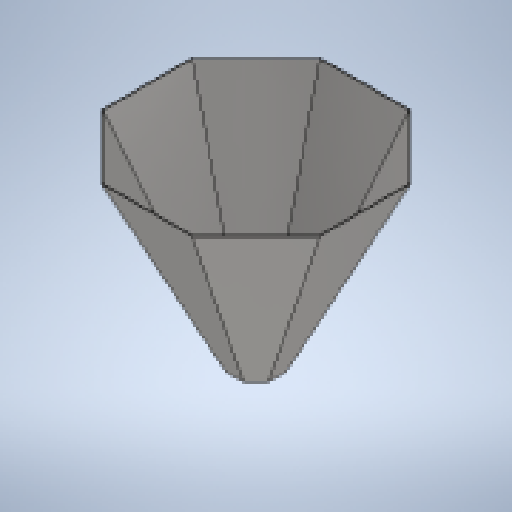
# Autodesk Inventor part: Funnel 1200x90 dummy
Saved by Autodesk Inventor 2025.1 (Build 291241020, 241B)
## iProperties
Created: 2025-07-11
Part Number: Funnel 1200x90 dummy
Material: Stainless Steel
Document SubType Name: Modeling
Designer: user
Density: 8 g/cm^3
Appearance: Semi-Polished
Author: user
Autodesk Inventor part; units mm, degrees
ref_plane "YZ Plane" through (0, 0, 0) normal (1, 0, 0) x (0, 1, 0)
ref_plane "XZ Plane" through (0, 0, 0) normal (0, 1, 0) x (-1, 0, 0)
ref_plane "XY Plane" through (0, 0, 0) normal (0, 0, 1) x (1, 0, 0)
sketch "Sketch1" plane through (0, 0, 0) normal (0, 0, 1) x (1, 0, 0)
  line L0 (18.6396, 45) -> (45, 18.6396)
  line L1 (45, 18.6396) -> (45, -18.6396)
  line L2 (45, -18.6396) -> (18.6396, -45)
  line L3 (18.6396, -45) -> (-18.6396, -45)
  line L4 (-18.6396, -45) -> (-45, -18.6396)
  line L5 (-45, -18.6396) -> (-45, 18.6396)
  line L6 (-45, 18.6396) -> (-18.6396, 45)
  line L7 (-18.6396, 45) -> (18.6396, 45)
  point P0 (0, 0)
  point P1 (0, 0)
  dimension "d0" = 90
  dimension "d1" = 37.2792
  constraints: 16 end point, 1 coincident, 1 vertical, 17 other
  measures "d0" distance between parallel lines of L3 L7
  measures "d1" distance of L6.end L0.start
extrude "Extrusion1" add sketch "Sketch1" along normal blind 400 draft 25
shell "Shell1" thickness 2 removed faces 2 at (31.9667, -77.1744, 400) at (-6.2132, -2.5736, 0)
body "Solid1"
